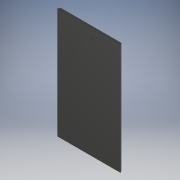
# Autodesk Inventor part: BA03
Saved by Autodesk Inventor 2017 (Build 210142000, 142)
## iProperties
Created: 2018-10-18
Part Number: BA03
Material: ABS Plastic
Document SubType Name: Modeling
Designer: Dell
Density: 1.06 g/cm^3
Appearance: Smooth - Black
Author: Dell
Autodesk Inventor part; units mm, degrees
ref_plane "YZ Plane" through (0, 0, 0) normal (1, 0, 0) x (0, 1, 0)
ref_plane "XZ Plane" through (0, 0, 0) normal (0, 1, 0) x (-1, 0, 0)
ref_plane "XY Plane" through (0, 0, 0) normal (0, 0, 1) x (1, 0, 0)
sketch "Sketch1" plane through (0, 0, 0) normal (0, 0, 1) x (1, 0, 0)
  line L0 (0, 0) -> (292.1, 0)
  line L1 (292.1, 0) -> (292.1, -533.4)
  line L2 (292.1, -533.4) -> (0, -533.4)
  line L3 (0, -533.4) -> (0, 0)
  dimension "d0" = 292.1
  dimension "d1" = 533.4
  constraints: 8 end point, 2 parallel, 1 horizontal, 1 perpendicular
  measures "d0" distance of L1.end L2.end
  measures "d1" distance of L0.end L1.end
extrude "Extrusion1" add sketch "Sketch1" along normal blind 10
sketch "Sketch2" plane through (0, 0, 0) normal (0, 1, 0) x (1, 0, 0)
  line L0 (292.1, -10) -> (0, -10) projected
  line L1 (0, -10) -> (-5.7735, -10)
  line L2 (-5.7735, -10) -> (0, 0)
  line L3 (0, 0) -> (0, -10) projected
  line L4 (0, 0) -> (0, -10) projected
  line L5 (0, -10) -> (0, 0)
  line L6 (292.1, -10) -> (297.8735, -10)
  line L7 (292.1, 0) -> (292.1, -10) projected
  line L8 (297.8735, -10) -> (292.1, 0)
  line L9 (292.1, 0) -> (292.1, -10)
  dimension "d4" = 30
  dimension "d5" = 60
  constraints: 12 end point, 2 collinear, 2 horizontal
  measures "d4" angle of L3 L2
  measures "d5" angle of L6 L8
extrude "Extrusion2" add sketch "Sketch2" against normal blind 533.4
sketch "Sketch5" plane through (0, 0, 10) normal (0, 0, 1) x (1, 0, 0)
  circle A0 centre (101, -44.45) radius 2.3812
  circle A1 centre (164.5, -44.45) radius 2.3813
  line L0 (-5.7735, 0) -> (297.8735, 0) projected
  line L1 (-5.7735, 0) -> (-5.7735, -533.4) projected
  line L2 (0, -533.4) -> (0, 0) projected
  dimension "d18" = 4.7625
  dimension "d19" = 63.5
  dimension "d20" = 4.7625
  dimension "d21" = 44.45
  dimension "d23" = 101
  constraints: 2 centre point, 1 horizontal alignment
  measures "d18" diameter of A0
  measures "d19" distance of A0.centre A1.centre
  measures "d20" diameter of A1
  measures "d21" distance from line of L0 A0.centre
  measures "d23" distance from line of A0.centre L2
extrude "Extrusion4" cut sketch "Sketch5" against normal through all
body "Solid1"
